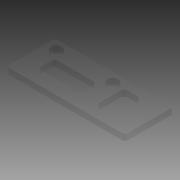
# Autodesk Inventor part: D-055
Saved by Autodesk Inventor 2015 (Build 190159000, 159)
## iProperties
Company: MARCHA TECHNOLOGY
Created: 2013-10-03
Part Number: D-055
Document SubType Name: Modeling
Designer: O.Martin
Density: 1 g/cm^3
Mass: 1.00024 g
Surface Area: 13.8644 cm^2
Volume: 1.00024 cm^3
Project: WITBOXprinter_K01
Description: SUPLEMENTO AISLANTE MICRO
Stock Number: 28655
Material: Generic
Appearance: Clear - Light
Author: O.Martin
Autodesk Inventor part; units mm, degrees
ref_plane "YZ Plane" through (0, 0, 0) normal (1, 0, 0) x (0, 1, 0)
ref_plane "XZ Plane" through (0, 0, 0) normal (0, 1, 0) x (-1, 0, 0)
ref_plane "XY Plane" through (0, 0, 0) normal (0, 0, 1) x (1, 0, 0)
sketch "Boceto1" plane through (0, 0, 0) normal (0, 0, 1) x (1, 0, 0)
  line L0 (-9, 12.2) -> (-9, 10.2) construction
  line L1 (-9, 10.2) -> (-12.5, 10.2) construction
  line L2 (-12.5, 10.2) -> (-12.5, 12.2) construction
  line L3 (-12.5, 12.2) -> (-9, 12.2) construction
  line L4 (-9, 7.2) -> (-9, 5.2) construction
  line L5 (-9, 5.2) -> (-12.5, 5.2) construction
  line L6 (-12.5, 5.2) -> (-12.5, 7.2) construction
  line L7 (-12.5, 7.2) -> (-9, 7.2) construction
  line L8 (-9, 9.7) -> (-9, 7.7) construction
  line L9 (-9, 7.7) -> (-12.5, 7.7) construction
  line L10 (-12.5, 7.7) -> (-12.5, 9.7) construction
  line L11 (-12.5, 9.7) -> (-9, 9.7) construction
  line L12 (-20.7, 9.2) -> (-20.7, 5.7) construction
  line L13 (-20.7, 5.7) -> (-22.7, 5.7) construction
  line L14 (-22.7, 5.7) -> (-22.7, 9.2) construction
  line L15 (-22.7, 9.2) -> (-20.7, 9.2) construction
  line L16 (-30.7, 9.2) -> (-30.7, 5.7) construction
  line L17 (-30.7, 5.7) -> (-32.7, 5.7) construction
  line L18 (-32.7, 5.7) -> (-32.7, 9.2) construction
  line L19 (-32.7, 9.2) -> (-30.7, 9.2) construction
  line L20 (-25.7, 9.2) -> (-25.7, 5.7) construction
  line L21 (-25.7, 5.7) -> (-27.7, 5.7) construction
  line L22 (-27.7, 5.7) -> (-27.7, 9.2) construction
  line L23 (-27.7, 9.2) -> (-25.7, 9.2) construction
  line L24 (0, 16.2) -> (0, 0) projected
  line L25 (-39.5, 16.2) -> (0, 16.2) projected
  line L26 (-39.5, 0) -> (-39.5, 16.2) projected
  line L27 (0, 0) -> (-39.5, 0) projected
  circle A0 centre (-36, 13.2) radius 1.5 projected
  circle A1 centre (-17.25, 13.2) radius 1.5 projected
  line L28 (-33.7, 10.2) -> (-19.7, 10.2)
  line L29 (-19.7, 10.2) -> (-19.7, 4.7)
  line L30 (-19.7, 4.7) -> (-33.7, 4.7)
  line L31 (-33.7, 4.7) -> (-33.7, 10.2)
  line L32 (-13.5, 13.2) -> (-8, 13.2)
  line L33 (-8, 13.2) -> (-8, 4.2)
  line L34 (-8, 4.2) -> (-13.5, 4.2)
  line L35 (-13.5, 4.2) -> (-13.5, 13.2)
  circle A2 centre (-36, 13.2) radius 2.0235
  circle A3 centre (-17.25, 13.2) radius 2.0407
  dimension "d0" = 1
  dimension "d1" = 1
  dimension "d2" = 1
  dimension "d3" = 1
  dimension "d4" = 1
  dimension "d5" = 1
  dimension "d6" = 1
  dimension "d7" = 1
  dimension "d11" = 4.047
  constraints: 16 end point, 4 parallel, 2 centre point, 2 coincident, 2 horizontal, 2 perpendicular
  measures "d0" distance between parallel lines of L18 L31
  measures "d1" distance between parallel lines of L29 L12
  measures "d2" distance between parallel lines of L28 L19
  measures "d3" distance between parallel lines of L30 L17
  measures "d4" distance between parallel lines of L32 L3
  measures "d5" distance between parallel lines of L5 L34
  measures "d6" distance between parallel lines of L33 L8
  measures "d7" distance between parallel lines of L35 L10
  measures "d11" diameter of A2
extrude "Extrusión1" add sketch "Boceto1" along normal blind 2 contours L24 L27 L26 L25 | A2 | A3
fillet "Empalme1" radius 1 12 edges at (-39.5, 16.2, 1) (-39.5, 0, 1) (0, 0, 1) (0, 16.2, 1) (-33.7, 10.2, 1) (-33.7, 4.7, 1) (-19.7, 4.7, 1) (-19.7, 10.2, 1) (-13.5, 13.2, 1) (-8, 13.2, 1) (-8, 4.2, 1) (-13.5, 4.2, 1)
sketch "Boceto2" plane through (0, 0, 2) normal (0, 0, 1) x (1, 0, 0)
  circle A0 centre (-17.25, 13.2) radius 1.5 projected
  circle A1 centre (-36, 13.2) radius 1.5 projected
  constraints: 2 coincident
hole "Agujero1" at (-36, 13.2, 2) at (-17.25, 13.2, 2) direction (0, 0, -1) diameter 3.5 depth 8 tip angle 118
equation "\"d1\" = d0"
equation "\"d2\" = d0"
equation "\"d3\" = d0"
equation "\"d4\" = d2"
equation "\"d5\" = d4"
equation "\"d6\" = d4"
equation "\"d7\" = d4"
body "Solid1"
